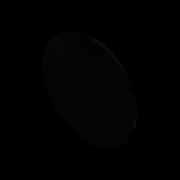
# Autodesk Inventor part: Plastic Plug
Saved by Autodesk Inventor 2014 SP1 (Build 180222100, 222)
## iProperties
Created: 2013-11-29
Part Number: Plastic Plug
Material: Plastic, Opaque Black
Document SubType Name: Modeling
Designer: Rauhul Varma
Mass: 2.59251 g
Surface Area: 41.7704 cm^2
Volume: 2.72322 cm^3
Density: 0.952 g/cm^3
Appearance: Smooth - Black
Author: Rauhul Varma
Autodesk Inventor part; units mm, degrees
ref_plane "YZ Plane" through (0, 0, 0) normal (1, 0, 0) x (0, 1, 0)
ref_plane "XZ Plane" through (0, 0, 0) normal (0, 1, 0) x (-1, 0, 0)
ref_plane "XY Plane" through (0, 0, 0) normal (0, 0, 1) x (1, 0, 0)
sketch "Sketch1" plane through (0, 0, 0) normal (0, 0, 1) x (1, 0, 0)
  circle A0 centre (0, 0) radius 20.6375
  circle A1 centre (0, 0) radius 17.4625
  dimension "d0" = 41.275
  dimension "d1" = 34.925
  constraints: 2 centre point, 2 coincident
  measures "d0" diameter of A0
  measures "d1" diameter of A1
extrude "Extrusion1" add sketch "Sketch1" along normal blind 1.5875
sketch "Sketch2" plane through (0, 0, 1.5875) normal (0, 0, 1) x (1, 0, 0)
  circle A0 centre (0, 0) radius 17.4625 projected
  circle A1 centre (0, 0) radius 20.6375 projected
  circle A2 centre (0, 0) radius 19.05
  dimension "d4" = 38.1
  constraints: 1 centre point, 1 coincident
  measures "d4" diameter of A2
extrude "Extrusion2" add sketch "Sketch2" along normal blind 1.5875 contours A2
sketch "Sketch3" plane through (0, 0, 3.175) normal (0, 0, 1) x (1, 0, 0)
  circle A0 centre (0, 0) radius 19.05 projected
  circle A1 centre (0, 0) radius 22.225
  dimension "d7" = 44.45
  constraints: 1 centre point, 1 coincident
  measures "d7" diameter of A1
extrude "Extrusion3" add sketch "Sketch3" along normal blind 1.5875 contours A0 | A1
chamfer "Chamfer1" distance 4.7625 distance2 1.5875 1 edges at (-22.225, 0, 4.7625) measured on face at (-21.725, 0, 4.7625)
chamfer "Chamfer2" distance 1.5875 angle 45 1 edges at (-17.4625, 0, 0)
body "Solid1"
